minecraftdiamondsword big CNC rotated_v6 (Autodesk Fusion 360 design; units mm, degrees)
Autodesk Fusion 360 part; units mm, degrees
sketch "big huge diamond sword" plane through (0, 0, 0) normal (0, 0, 1) x (1, 0, 0)
  line L0 (0, 62.2254) -> (7.7782, 54.4472)
  line L1 (7.7782, 54.4472) -> (15.5563, 62.2254)
  line L2 (15.5563, 62.2254) -> (7.7782, 70.0036)
  line L3 (7.7782, 70.0036) -> (0, 62.2254)
  line L4 (7.7782, 54.4472) -> (15.5563, 46.669)
  line L5 (15.5563, 46.669) -> (23.3345, 54.4472)
  line L6 (23.3345, 54.4472) -> (15.5563, 62.2254)
  line L7 (15.5563, 62.2254) -> (7.7782, 54.4472)
  line L8 (15.5563, 46.669) -> (23.3345, 38.8909)
  line L9 (23.3345, 38.8909) -> (31.1127, 46.669)
  line L10 (23.3345, 54.4472) -> (15.5563, 46.669)
  line L11 (7.7782, 70.0036) -> (15.5563, 62.2254)
  line L12 (15.5563, 62.2254) -> (23.3345, 70.0036)
  line L13 (23.3345, 70.0036) -> (15.5563, 77.7817)
  line L14 (15.5563, 77.7817) -> (7.7782, 70.0036)
  line L15 (23.3345, 70.0036) -> (31.1127, 62.2254)
  line L16 (31.1127, 62.2254) -> (23.3345, 54.4472)
  line L17 (23.3345, 54.4472) -> (15.5563, 62.2254)
  line L18 (15.5563, 62.2254) -> (23.3345, 70.0036)
  line L19 (15.5563, 77.7817) -> (23.3345, 70.0036)
  line L20 (23.3345, 70.0036) -> (31.1127, 77.7817)
  line L21 (31.1127, 77.7817) -> (23.3345, 85.5599)
  line L22 (23.3345, 85.5599) -> (15.5563, 77.7817)
  line L23 (23.3345, 70.0036) -> (31.1127, 62.2254)
  line L24 (31.1127, 62.2254) -> (38.8909, 70.0036)
  line L25 (38.8909, 70.0036) -> (31.1127, 77.7817)
  line L26 (31.1127, 77.7817) -> (23.3345, 70.0036)
  line L27 (31.1127, 62.2254) -> (38.8909, 54.4472)
  line L28 (38.8909, 54.4472) -> (31.1127, 46.669)
  line L29 (31.1127, 46.669) -> (23.3345, 54.4472)
  line L30 (23.3345, 54.4472) -> (31.1127, 62.2254)
  line L31 (31.1127, 62.2254) -> (38.8909, 54.4472)
  line L32 (38.8909, 54.4472) -> (46.669, 62.2254)
  line L33 (46.669, 62.2254) -> (38.8909, 70.0036)
  line L34 (38.8909, 70.0036) -> (31.1127, 62.2254)
  line L35 (38.8909, 70.0036) -> (46.669, 62.2254)
  line L36 (46.669, 62.2254) -> (54.4472, 70.0036)
  line L37 (54.4472, 70.0036) -> (46.669, 77.7817)
  line L38 (46.669, 77.7817) -> (38.8909, 70.0036)
  line L39 (46.669, 62.2254) -> (54.4472, 54.4472)
  line L40 (54.4472, 54.4472) -> (46.669, 46.669)
  line L41 (46.669, 46.669) -> (38.8909, 54.4472)
  line L42 (38.8909, 54.4472) -> (46.669, 62.2254)
  line L43 (46.669, 62.2254) -> (54.4472, 54.4472)
  line L44 (54.4472, 54.4472) -> (62.2254, 62.2254)
  line L45 (62.2254, 62.2254) -> (54.4472, 70.0036)
  line L46 (54.4472, 70.0036) -> (46.669, 62.2254)
  line L47 (54.4472, 70.0036) -> (62.2254, 62.2254)
  line L48 (62.2254, 62.2254) -> (70.0036, 70.0036)
  line L49 (70.0036, 70.0036) -> (62.2254, 77.7817)
  line L50 (62.2254, 77.7817) -> (54.4472, 70.0036)
  line L51 (62.2254, 62.2254) -> (70.0036, 54.4472)
  line L52 (62.2254, 46.669) -> (54.4472, 54.4472)
  line L53 (54.4472, 54.4472) -> (62.2254, 62.2254)
  line L54 (62.2254, 62.2254) -> (70.0036, 54.4472)
  line L55 (70.0036, 54.4472) -> (77.7817, 62.2254)
  line L56 (77.7817, 62.2254) -> (70.0036, 70.0036)
  line L57 (70.0036, 70.0036) -> (62.2254, 62.2254)
  line L58 (70.0036, 70.0036) -> (77.7817, 62.2254)
  line L59 (77.7817, 62.2254) -> (85.5599, 70.0036)
  line L60 (85.5599, 70.0036) -> (77.7817, 77.7817)
  line L61 (77.7817, 77.7817) -> (70.0036, 70.0036)
  line L62 (77.7817, 77.7817) -> (70.0036, 85.5599)
  line L63 (70.0036, 85.5599) -> (77.7817, 93.3381)
  line L64 (77.7817, 93.3381) -> (85.5599, 85.5599)
  line L65 (85.5599, 85.5599) -> (77.7817, 77.7817)
  line L66 (77.7817, 93.3381) -> (85.5599, 85.5599)
  line L67 (85.5599, 85.5599) -> (93.3381, 93.3381)
  line L68 (93.3381, 93.3381) -> (85.5599, 101.1163)
  line L69 (85.5599, 101.1163) -> (77.7817, 93.3381)
  line L70 (85.5599, 101.1163) -> (77.7817, 108.8944)
  line L71 (77.7817, 108.8944) -> (85.5599, 116.6726)
  line L72 (85.5599, 116.6726) -> (93.3381, 108.8944)
  line L73 (93.3381, 108.8944) -> (85.5599, 101.1163)
  line L74 (85.5599, 116.6726) -> (93.3381, 108.8944)
  line L75 (93.3381, 108.8944) -> (101.1163, 116.6726)
  line L76 (101.1163, 116.6726) -> (93.3381, 124.4508)
  line L77 (93.3381, 124.4508) -> (85.5599, 116.6726)
  line L78 (93.3381, 108.8944) -> (101.1163, 101.1163)
  line L79 (101.1163, 101.1163) -> (108.8944, 108.8944)
  line L80 (108.8944, 108.8944) -> (101.1163, 116.6726)
  line L81 (101.1163, 116.6726) -> (93.3381, 108.8944)
  line L82 (85.5599, 101.1163) -> (93.3381, 93.3381)
  line L83 (93.3381, 93.3381) -> (101.1163, 101.1163)
  line L84 (101.1163, 101.1163) -> (93.3381, 108.8944)
  line L85 (93.3381, 108.8944) -> (85.5599, 101.1163)
  line L86 (101.1163, 101.1163) -> (108.8944, 93.3381)
  line L87 (108.8944, 93.3381) -> (101.1163, 85.5599)
  line L88 (101.1163, 85.5599) -> (93.3381, 93.3381)
  line L89 (93.3381, 93.3381) -> (101.1163, 101.1163)
  line L90 (93.3381, 93.3381) -> (101.1163, 85.5599)
  line L91 (101.1163, 85.5599) -> (93.3381, 77.7817)
  line L92 (93.3381, 77.7817) -> (85.5599, 85.5599)
  line L93 (85.5599, 85.5599) -> (93.3381, 93.3381)
  line L94 (77.7817, 77.7817) -> (85.5599, 70.0036)
  line L95 (85.5599, 70.0036) -> (93.3381, 77.7817)
  line L96 (93.3381, 77.7817) -> (85.5599, 85.5599)
  line L97 (85.5599, 85.5599) -> (77.7817, 77.7817)
  line L98 (70.0036, 54.4472) -> (77.7817, 46.669)
  line L99 (62.2254, 46.669) -> (70.0036, 54.4472)
  line L100 (77.7817, 62.2254) -> (85.5599, 54.4472)
  line L101 (85.5599, 54.4472) -> (77.7817, 46.669)
  line L102 (70.0036, 54.4472) -> (77.7817, 62.2254)
  line L103 (85.5599, 70.0036) -> (93.3381, 62.2254)
  line L104 (93.3381, 62.2254) -> (85.5599, 54.4472)
  line L105 (85.5599, 54.4472) -> (77.7817, 62.2254)
  line L106 (77.7817, 62.2254) -> (85.5599, 70.0036)
  line L107 (77.7817, 46.669) -> (85.5599, 38.8909)
  line L108 (85.5599, 38.8909) -> (77.7817, 31.1127)
  line L109 (77.7817, 31.1127) -> (70.0036, 38.8909)
  line L110 (70.0036, 38.8909) -> (77.7817, 46.669)
  line L111 (77.7817, 46.669) -> (85.5599, 38.8909)
  line L112 (85.5599, 38.8909) -> (93.3381, 46.669)
  line L113 (93.3381, 46.669) -> (85.5599, 54.4472)
  line L114 (85.5599, 54.4472) -> (77.7817, 46.669)
  line L115 (85.5599, 38.8909) -> (93.3381, 31.1127)
  line L116 (93.3381, 31.1127) -> (85.5599, 23.3345)
  line L117 (85.5599, 23.3345) -> (77.7817, 31.1127)
  line L118 (77.7817, 31.1127) -> (85.5599, 38.8909)
  line L119 (85.5599, 23.3345) -> (93.3381, 15.5563)
  line L120 (93.3381, 15.5563) -> (101.1163, 23.3345)
  line L121 (101.1163, 23.3345) -> (93.3381, 31.1127)
  line L122 (93.3381, 31.1127) -> (85.5599, 23.3345)
  line L123 (93.3381, 15.5563) -> (101.1163, 7.7782)
  line L124 (101.1163, 7.7782) -> (108.8944, 15.5563)
  line L125 (108.8944, 15.5563) -> (101.1163, 23.3345)
  line L126 (101.1163, 23.3345) -> (93.3381, 15.5563)
  line L127 (85.5599, 23.3345) -> (93.3381, 15.5563)
  line L128 (93.3381, 15.5563) -> (85.5599, 7.7782)
  line L129 (85.5599, 7.7782) -> (77.7817, 15.5563)
  line L130 (77.7817, 15.5563) -> (85.5599, 23.3345)
  line L131 (93.3381, 15.5563) -> (101.1163, 7.7782)
  line L132 (101.1163, 7.7782) -> (93.3381, 0)
  line L133 (93.3381, 0) -> (85.5599, 7.7782)
  line L134 (85.5599, 7.7782) -> (93.3381, 15.5563)
  line L135 (93.3381, 77.7817) -> (101.1163, 70.0036)
  line L136 (101.1163, 70.0036) -> (93.3381, 62.2254)
  line L137 (93.3381, 62.2254) -> (85.5599, 70.0036)
  line L138 (85.5599, 70.0036) -> (93.3381, 77.7817)
  line L139 (93.3381, 62.2254) -> (101.1163, 54.4472)
  line L140 (101.1163, 54.4472) -> (93.3381, 46.669)
  line L141 (93.3381, 46.669) -> (85.5599, 54.4472)
  line L142 (85.5599, 54.4472) -> (93.3381, 62.2254)
  line L143 (101.1163, 85.5599) -> (108.8944, 77.7817)
  line L144 (108.8944, 77.7817) -> (101.1163, 70.0036)
  line L145 (101.1163, 70.0036) -> (93.3381, 77.7817)
  line L146 (93.3381, 77.7817) -> (101.1163, 85.5599)
  line L147 (101.1163, 70.0036) -> (108.8944, 62.2254)
  line L148 (108.8944, 62.2254) -> (101.1163, 54.4472)
  line L149 (101.1163, 54.4472) -> (93.3381, 62.2254)
  line L150 (93.3381, 62.2254) -> (101.1163, 70.0036)
  line L151 (108.8944, 77.7817) -> (116.6726, 70.0036)
  line L152 (116.6726, 70.0036) -> (108.8944, 62.2254)
  line L153 (108.8944, 62.2254) -> (101.1163, 70.0036)
  line L154 (101.1163, 70.0036) -> (108.8944, 77.7817)
  line L155 (93.3381, 46.669) -> (101.1163, 38.8909)
  line L156 (101.1163, 38.8909) -> (93.3381, 31.1127)
  line L157 (93.3381, 31.1127) -> (85.5599, 38.8909)
  line L158 (85.5599, 38.8909) -> (93.3381, 46.669)
  line L159 (101.1163, 38.8909) -> (108.8944, 31.1127)
  line L160 (108.8944, 31.1127) -> (101.1163, 23.3345)
  line L161 (101.1163, 23.3345) -> (93.3381, 31.1127)
  line L162 (93.3381, 31.1127) -> (101.1163, 38.8909)
  line L163 (101.1163, 54.4472) -> (108.8944, 46.669)
  line L164 (108.8944, 46.669) -> (101.1163, 38.8909)
  line L165 (101.1163, 38.8909) -> (93.3381, 46.669)
  line L166 (93.3381, 46.669) -> (101.1163, 54.4472)
  line L167 (108.8944, 62.2254) -> (116.6726, 54.4472)
  line L168 (116.6726, 54.4472) -> (108.8944, 46.669)
  line L169 (108.8944, 46.669) -> (101.1163, 54.4472)
  line L170 (101.1163, 54.4472) -> (108.8944, 62.2254)
  line L171 (108.8944, 46.669) -> (101.1163, 54.4472)
  line L172 (101.1163, 54.4472) -> (108.8944, 62.2254)
  line L173 (108.8944, 62.2254) -> (116.6726, 54.4472)
  line L174 (116.6726, 54.4472) -> (108.8944, 46.669)
  line L175 (108.8944, 46.669) -> (116.6726, 38.8909)
  line L176 (116.6726, 38.8909) -> (124.4508, 46.669)
  line L177 (124.4508, 46.669) -> (116.6726, 54.4472)
  line L178 (116.6726, 54.4472) -> (108.8944, 46.669)
  line L179 (108.8944, 62.2254) -> (116.6726, 54.4472)
  line L180 (116.6726, 54.4472) -> (124.4508, 62.2254)
  line L181 (124.4508, 62.2254) -> (116.6726, 70.0036)
  line L182 (116.6726, 70.0036) -> (108.8944, 62.2254)
  line L183 (116.6726, 54.4472) -> (124.4508, 46.669)
  line L184 (124.4508, 46.669) -> (132.229, 54.4472)
  line L185 (132.229, 54.4472) -> (124.4508, 62.2254)
  line L186 (124.4508, 62.2254) -> (116.6726, 54.4472)
  line L187 (124.4508, 46.669) -> (132.229, 38.8909)
  line L188 (132.229, 38.8909) -> (140.0071, 46.669)
  line L189 (140.0071, 46.669) -> (132.229, 54.4472)
  line L190 (132.229, 54.4472) -> (124.4508, 46.669)
  line L191 (108.8944, 77.7817) -> (116.6726, 70.0036)
  line L192 (116.6726, 70.0036) -> (124.4508, 77.7817)
  line L193 (124.4508, 77.7817) -> (116.6726, 85.5599)
  line L194 (116.6726, 85.5599) -> (108.8944, 77.7817)
  line L195 (116.6726, 70.0036) -> (124.4508, 62.2254)
  line L196 (124.4508, 62.2254) -> (132.229, 70.0036)
  line L197 (132.229, 70.0036) -> (124.4508, 77.7817)
  line L198 (124.4508, 77.7817) -> (116.6726, 70.0036)
  line L199 (132.229, 70.0036) -> (124.4508, 77.7817)
  line L200 (124.4508, 77.7817) -> (132.229, 85.5599)
  line L201 (132.229, 85.5599) -> (140.0071, 77.7817)
  line L202 (140.0071, 77.7817) -> (132.229, 70.0036)
  line L203 (124.4508, 62.2254) -> (132.229, 54.4472)
  line L204 (132.229, 54.4472) -> (140.0071, 62.2254)
  line L205 (140.0071, 62.2254) -> (132.229, 70.0036)
  line L206 (132.229, 70.0036) -> (124.4508, 62.2254)
  line L207 (132.229, 70.0036) -> (140.0071, 62.2254)
  line L208 (140.0071, 62.2254) -> (147.7853, 70.0036)
  line L209 (147.7853, 70.0036) -> (140.0071, 77.7817)
  line L210 (140.0071, 77.7817) -> (132.229, 70.0036)
  line L211 (132.229, 54.4472) -> (140.0071, 46.669)
  line L212 (140.0071, 46.669) -> (147.7853, 54.4472)
  line L213 (147.7853, 54.4472) -> (140.0071, 62.2254)
  line L214 (140.0071, 62.2254) -> (132.229, 54.4472)
  line L215 (140.0071, 77.7817) -> (147.7853, 70.0036)
  line L216 (147.7853, 70.0036) -> (155.5635, 77.7817)
  line L217 (155.5635, 77.7817) -> (147.7853, 85.5599)
  line L218 (147.7853, 85.5599) -> (140.0071, 77.7817)
  line L219 (140.0071, 46.669) -> (147.7853, 38.8909)
  line L220 (147.7853, 38.8909) -> (155.5635, 46.669)
  line L221 (155.5635, 46.669) -> (147.7853, 54.4472)
  line L222 (147.7853, 54.4472) -> (140.0071, 46.669)
  line L223 (140.0071, 62.2254) -> (147.7853, 54.4472)
  line L224 (147.7853, 54.4472) -> (155.5635, 62.2254)
  line L225 (155.5635, 62.2254) -> (147.7853, 70.0036)
  line L226 (147.7853, 70.0036) -> (140.0071, 62.2254)
  line L227 (155.5635, 62.2254) -> (163.3417, 54.4472)
  line L228 (163.3417, 54.4472) -> (171.1198, 62.2254)
  line L229 (171.1198, 62.2254) -> (163.3417, 70.0036)
  line L230 (163.3417, 70.0036) -> (155.5635, 62.2254)
  line L231 (155.5635, 62.2254) -> (147.7853, 70.0036)
  line L232 (147.7853, 70.0036) -> (155.5635, 77.7817)
  line L233 (155.5635, 77.7817) -> (163.3417, 70.0036)
  line L234 (163.3417, 70.0036) -> (155.5635, 62.2254)
  line L235 (155.5635, 62.2254) -> (163.3417, 54.4472)
  line L236 (163.3417, 54.4472) -> (155.5635, 46.669)
  line L237 (155.5635, 46.669) -> (147.7853, 54.4472)
  line L238 (147.7853, 54.4472) -> (155.5635, 62.2254)
  line L239 (155.5635, 77.7817) -> (163.3417, 70.0036)
  line L240 (163.3417, 70.0036) -> (171.1198, 77.7817)
  line L241 (171.1198, 77.7817) -> (163.3417, 85.5599)
  line L242 (163.3417, 85.5599) -> (155.5635, 77.7817)
  line L243 (163.3417, 70.0036) -> (171.1198, 62.2254)
  line L244 (171.1198, 62.2254) -> (178.898, 70.0036)
  line L245 (178.898, 70.0036) -> (171.1198, 77.7817)
  line L246 (171.1198, 77.7817) -> (163.3417, 70.0036)
  line L247 (155.5635, 46.669) -> (163.3417, 38.8909)
  line L248 (163.3417, 38.8909) -> (171.1198, 46.669)
  line L249 (171.1198, 46.669) -> (163.3417, 54.4472)
  line L250 (163.3417, 54.4472) -> (155.5635, 46.669)
  line L251 (163.3417, 54.4472) -> (171.1198, 46.669)
  line L252 (171.1198, 46.669) -> (178.898, 54.4472)
  line L253 (178.898, 54.4472) -> (171.1198, 62.2254)
  line L254 (171.1198, 62.2254) -> (163.3417, 54.4472)
  line L255 (171.1198, 62.2254) -> (178.898, 54.4472)
  line L256 (178.898, 54.4472) -> (186.6762, 62.2254)
  line L257 (186.6762, 62.2254) -> (178.898, 70.0036)
  line L258 (178.898, 70.0036) -> (171.1198, 62.2254)
  line L259 (171.1198, 77.7817) -> (178.898, 70.0036)
  line L260 (178.898, 70.0036) -> (186.6762, 77.7817)
  line L261 (186.6762, 77.7817) -> (178.898, 85.5599)
  line L262 (178.898, 85.5599) -> (171.1198, 77.7817)
  line L263 (171.1198, 46.669) -> (178.898, 38.8909)
  line L264 (178.898, 38.8909) -> (186.6762, 46.669)
  line L265 (186.6762, 46.669) -> (178.898, 54.4472)
  line L266 (178.898, 54.4472) -> (171.1198, 46.669)
  line L267 (178.898, 70.0036) -> (186.6762, 62.2254)
  line L268 (186.6762, 62.2254) -> (194.4544, 70.0036)
  line L269 (194.4544, 70.0036) -> (186.6762, 77.7817)
  line L270 (186.6762, 77.7817) -> (178.898, 70.0036)
  line L271 (178.898, 54.4472) -> (186.6762, 46.669)
  line L272 (186.6762, 46.669) -> (194.4544, 54.4472)
  line L273 (194.4544, 54.4472) -> (186.6762, 62.2254)
  line L274 (186.6762, 62.2254) -> (178.898, 54.4472)
  line L275 (186.6762, 62.2254) -> (194.4544, 54.4472)
  line L276 (194.4544, 54.4472) -> (202.2325, 62.2254)
  line L277 (202.2325, 62.2254) -> (194.4544, 70.0036)
  line L278 (194.4544, 70.0036) -> (186.6762, 62.2254)
  line L279 (186.6762, 46.669) -> (194.4544, 38.8909)
  line L280 (194.4544, 38.8909) -> (202.2325, 46.669)
  line L281 (202.2325, 46.669) -> (194.4544, 54.4472)
  line L282 (194.4544, 54.4472) -> (186.6762, 46.669)
  line L283 (186.6762, 77.7817) -> (194.4544, 70.0036)
  line L284 (194.4544, 70.0036) -> (202.2325, 77.7817)
  line L285 (202.2325, 77.7817) -> (194.4544, 85.5599)
  line L286 (194.4544, 85.5599) -> (186.6762, 77.7817)
  line L287 (202.2325, 62.2254) -> (210.0107, 54.4472)
  line L288 (210.0107, 54.4472) -> (202.2325, 46.669)
  line L289 (202.2325, 46.669) -> (194.4544, 54.4472)
  line L290 (194.4544, 54.4472) -> (202.2325, 62.2254)
  line L291 (194.4544, 70.0036) -> (202.2325, 62.2254)
  line L292 (202.2325, 62.2254) -> (210.0107, 70.0036)
  line L293 (210.0107, 70.0036) -> (202.2325, 77.7817)
  line L294 (202.2325, 77.7817) -> (194.4544, 70.0036)
  line L295 (202.2325, 62.2254) -> (210.0107, 54.4472)
  line L296 (210.0107, 54.4472) -> (217.7889, 62.2254)
  line L297 (217.7889, 62.2254) -> (210.0107, 70.0036)
  line L298 (210.0107, 70.0036) -> (202.2325, 62.2254)
  line L299 (202.2325, 46.669) -> (210.0107, 38.8909)
  line L300 (210.0107, 38.8909) -> (217.7889, 46.669)
  line L301 (217.7889, 46.669) -> (210.0107, 54.4472)
  line L302 (210.0107, 54.4472) -> (202.2325, 46.669)
  line L303 (202.2325, 77.7817) -> (210.0107, 70.0036)
  line L304 (210.0107, 70.0036) -> (217.7889, 77.7817)
  line L305 (217.7889, 77.7817) -> (210.0107, 85.5599)
  line L306 (210.0107, 85.5599) -> (202.2325, 77.7817)
  line L307 (217.7889, 77.7817) -> (225.5671, 70.0036)
  line L308 (225.5671, 70.0036) -> (217.7889, 62.2254)
  line L309 (217.7889, 62.2254) -> (210.0107, 70.0036)
  line L310 (210.0107, 70.0036) -> (217.7889, 77.7817)
  line L311 (210.0107, 54.4472) -> (217.7889, 46.669)
  line L312 (217.7889, 46.669) -> (225.5671, 54.4472)
  line L313 (225.5671, 54.4472) -> (217.7889, 62.2254)
  line L314 (217.7889, 62.2254) -> (210.0107, 54.4472)
  line L315 (217.7889, 62.2254) -> (225.5671, 54.4472)
  line L316 (225.5671, 54.4472) -> (233.3452, 62.2254)
  line L317 (233.3452, 62.2254) -> (225.5671, 70.0036)
  line L318 (225.5671, 70.0036) -> (217.7889, 62.2254)
  line L319 (217.7889, 77.7817) -> (225.5671, 70.0036)
  line L320 (225.5671, 70.0036) -> (233.3452, 77.7817)
  line L321 (233.3452, 77.7817) -> (225.5671, 85.5599)
  line L322 (225.5671, 85.5599) -> (217.7889, 77.7817)
  line L323 (225.5671, 70.0036) -> (233.3452, 62.2254)
  line L324 (233.3452, 62.2254) -> (241.1234, 70.0036)
  line L325 (241.1234, 70.0036) -> (233.3452, 77.7817)
  line L326 (233.3452, 77.7817) -> (225.5671, 70.0036)
  line L327 (217.7889, 46.669) -> (225.5671, 38.8909)
  line L328 (225.5671, 38.8909) -> (233.3452, 46.669)
  line L329 (233.3452, 46.669) -> (225.5671, 54.4472)
  line L330 (225.5671, 54.4472) -> (217.7889, 46.669)
  line L331 (225.5671, 54.4472) -> (233.3452, 46.669)
  line L332 (233.3452, 46.669) -> (241.1234, 54.4472)
  line L333 (241.1234, 54.4472) -> (233.3452, 62.2254)
  line L334 (233.3452, 62.2254) -> (225.5671, 54.4472)
  line L335 (233.3452, 62.2254) -> (225.5671, 70.0036)
  line L336 (225.5671, 70.0036) -> (233.3452, 77.7817)
  line L337 (233.3452, 77.7817) -> (241.1234, 70.0036)
  line L338 (241.1234, 70.0036) -> (233.3452, 62.2254)
  line L339 (233.3452, 62.2254) -> (241.1234, 54.4472)
  line L340 (241.1234, 54.4472) -> (248.9016, 62.2254)
  line L341 (248.9016, 62.2254) -> (241.1234, 70.0036)
  line L342 (241.1234, 70.0036) -> (233.3452, 62.2254)
  circle A0 centre (10, 10) radius 2.05
  circle A1 centre (200, 10) radius 2.05
  line L343 (0, 62.2254) -> (248.9016, 62.2254) construction
  circle A2 centre (200, 114.4508) radius 2.05
  point P0 (10, 114.4508)
  dimension "d249" = 11
  dimension "d250" = 11
  dimension "d251" = 11
  dimension "d252" = 11
  dimension "d253" = 11
  dimension "d254" = 11
  dimension "d255" = 11
  dimension "d256" = 11
  dimension "d261" = 11
  dimension "d262" = 11
  dimension "d263" = 11
  dimension "d264" = 11
  dimension "d265" = 11
  dimension "d266" = 11
  dimension "d267" = 11
  dimension "d268" = 11
  dimension "d271" = 11
  dimension "d272" = 11
  dimension "d273" = 11
  dimension "d274" = 11
  dimension "d275" = 11
  dimension "d276" = 11
  dimension "d277" = 11
  dimension "d278" = 11
  dimension "d279" = 11
  dimension "d280" = 11
  dimension "d281" = 11
  dimension "d282" = 11
  dimension "d283" = 11
  dimension "d284" = 11
  dimension "d285" = 11
  dimension "d286" = 11
  dimension "d287" = 11
  dimension "d288" = 11
  dimension "d289" = 11
  dimension "d290" = 11
  dimension "d291" = 11
  dimension "d292" = 11
  dimension "d293" = 11
  dimension "d294" = 11
  dimension "d295" = 11
  dimension "d296" = 11
  dimension "d297" = 11
  dimension "d298" = 11
  dimension "d299" = 11
  dimension "d300" = 11
  dimension "d301" = 11
  dimension "d302" = 11
  dimension "d303" = 11
  dimension "d304" = 11
  dimension "d309" = 11
  dimension "d310" = 11
  dimension "d311" = 11
  dimension "d312" = 11
  dimension "d313" = 11
  dimension "d314" = 11
  dimension "d315" = 11
  dimension "d316" = 11
  dimension "d319" = 11
  dimension "d320" = 11
  dimension "d321" = 11
  dimension "d322" = 11
  dimension "d323" = 11
  dimension "d324" = 11
  dimension "d325" = 11
  dimension "d326" = 11
  dimension "d327" = 11
  dimension "d328" = 11
  dimension "d329" = 11
  dimension "d330" = 11
  dimension "d331" = 11
  dimension "d332" = 11
  dimension "d333" = 11
  dimension "d334" = 11
  dimension "d335" = 11
  dimension "d336" = 11
  dimension "d337" = 11
  dimension "d338" = 11
  dimension "d339" = 11
  dimension "d340" = 11
  dimension "d341" = 11
  dimension "d342" = 11
  dimension "d343" = 11
  dimension "d344" = 11
  dimension "d345" = 11
  dimension "d346" = 11
  dimension "d347" = 11
  dimension "d348" = 11
  dimension "d349" = 11
  dimension "d350" = 11
  dimension "d351" = 11
  dimension "d352" = 11
  dimension "d353" = 11
  dimension "d354" = 11
  dimension "d355" = 11
  dimension "d356" = 11
  dimension "d357" = 11
  dimension "d358" = 11
  dimension "d359" = 11
  dimension "d360" = 11
  dimension "d361" = 11
  dimension "d362" = 11
  dimension "d363" = 11
  dimension "d364" = 11
  dimension "d365" = 11
  dimension "d366" = 11
  dimension "d367" = 11
  dimension "d368" = 11
  dimension "d369" = 11
  dimension "d370" = 11
  dimension "d371" = 11
  dimension "d372" = 11
  dimension "d373" = 11
  dimension "d374" = 11
  dimension "d375" = 11
  dimension "d376" = 11
  dimension "d377" = 11
  dimension "d378" = 11
  dimension "d379" = 11
  dimension "d380" = 11
  dimension "d381" = 11
  dimension "d382" = 11
  dimension "d383" = 11
  dimension "d384" = 11
  dimension "d385" = 11
  dimension "d386" = 11
  dimension "d387" = 11
  dimension "d388" = 11
  dimension "d389" = 11
  dimension "d390" = 11
  dimension "d391" = 11
  dimension "d392" = 11
  dimension "d393" = 11
  dimension "d394" = 11
  dimension "d395" = 11
  dimension "d396" = 11
  dimension "d397" = 11
  dimension "d398" = 11
  dimension "d399" = 11
  dimension "d400" = 11
  dimension "d401" = 11
  dimension "d402" = 11
  dimension "d403" = 11
  dimension "d404" = 11
  dimension "d405" = 11
  dimension "d406" = 11
  dimension "d407" = 11
  dimension "d408" = 11
  dimension "d409" = 11
  dimension "d410" = 11
  dimension "d411" = 11
  dimension "d412" = 11
  dimension "d413" = 11
  dimension "d414" = 11
  dimension "d415" = 11
  dimension "d416" = 11
  dimension "d417" = 11
  dimension "d418" = 11
  dimension "d419" = 11
  dimension "d420" = 11
  dimension "d421" = 11
  dimension "d422" = 11
  dimension "d423" = 11
  dimension "d424" = 11
  dimension "d425" = 11
  dimension "d426" = 11
  dimension "d427" = 11
  dimension "d428" = 11
  dimension "d429" = 11
  dimension "d430" = 11
  dimension "d431" = 11
  dimension "d432" = 11
  dimension "d433" = 11
  dimension "d434" = 11
  dimension "d453" = 4.1
  dimension "d454" = 4.1
  dimension "d455" = 10
  dimension "d456" = 200
  dimension "d457" = 10
  constraint perpendicular L74 L75
  constraint parallel L75 L77
  constraint perpendicular L78 L79
  constraint parallel L79 L81
  constraint perpendicular L86 L87
  constraint parallel L87 L89
  constraint perpendicular L103 L104
  constraint parallel L104 L106
  constraint perpendicular L52 L99
  constraint coincident L98.end L101.end
  constraint perpendicular L115 L116
  constraint parallel L116 L118
  constraint perpendicular L123 L124
  constraint parallel L124 L126
  constraint perpendicular L127 L128
  constraint parallel L128 L130
  constraint perpendicular L131 L132
  constraint parallel L132 L134
  constraint perpendicular L135 L136
  constraint parallel L136 L138
  constraint perpendicular L139 L140
  constraint parallel L140 L142
  constraint perpendicular L143 L144
  constraint parallel L144 L146
  constraint perpendicular L147 L148
  constraint parallel L148 L150
  constraint perpendicular L151 L152
  constraint parallel L152 L154
  constraint perpendicular L155 L156
  constraint parallel L156 L158
  constraint perpendicular L159 L160
  constraint parallel L160 L162
  constraint perpendicular L163 L164
  constraint parallel L164 L166
  constraint perpendicular L167 L168
  constraint parallel L168 L170
  constraint perpendicular L171 L172
  constraint parallel L172 L174
  constraint perpendicular L175 L176
  constraint parallel L176 L178
  constraint perpendicular L179 L180
  constraint parallel L180 L182
  constraint perpendicular L183 L184
  constraint parallel L184 L186
  constraint perpendicular L187 L188
  constraint parallel L188 L190
  constraint perpendicular L195 L196
  constraint parallel L196 L198
  constraint perpendicular L199 L200
  constraint parallel L200 L202
  constraint perpendicular L203 L204
  constraint parallel L204 L206
  constraint perpendicular L211 L212
  constraint parallel L212 L214
  constraint perpendicular L215 L216
  constraint parallel L216 L218
  constraint perpendicular L219 L220
  constraint parallel L220 L222
  constraint perpendicular L223 L224
  constraint parallel L224 L226
  constraint perpendicular L227 L228
  constraint parallel L228 L230
  constraint perpendicular L231 L232
  constraint parallel L232 L234
  constraint perpendicular L235 L236
  constraint parallel L236 L238
  constraint perpendicular L239 L240
  constraint parallel L240 L242
  constraint perpendicular L243 L244
  constraint parallel L244 L246
  constraint perpendicular L247 L248
  constraint parallel L248 L250
  constraint perpendicular L251 L252
  constraint parallel L252 L254
  constraint perpendicular L255 L256
  constraint parallel L256 L258
  constraint perpendicular L259 L260
  constraint parallel L260 L262
  constraint perpendicular L263 L264
  constraint parallel L264 L266
  constraint perpendicular L267 L268
  constraint parallel L268 L270
  constraint perpendicular L275 L276
  constraint parallel L276 L278
  constraint perpendicular L279 L280
  constraint parallel L280 L282
  constraint perpendicular L283 L284
  constraint parallel L284 L286
  constraint perpendicular L287 L288
  constraint parallel L288 L290
  constraint perpendicular L291 L292
  constraint parallel L292 L294
  constraint perpendicular L303 L304
  constraint parallel L304 L306
  constraint perpendicular L339 L340
  constraint parallel L340 L342
  constraint horizontal A0.centre A1.centre
  constraint symmetric A0.centre L343 P0
  constraint symmetric A1 L343 A2
  measures "d249" distance of L0.start L0.end
  measures "d250" distance of L0.start L2.end
  measures "d251" distance of L0.end L4.end
  measures "d252" distance of L0.end L1.end
  measures "d253" distance of L4.end L8.end
  measures "d254" distance of L4.end L5.end
  measures "d255" distance of L2.end L1.end
  measures "d256" distance of L2.end L13.end
  measures "d261" distance of L12.end L15.end
  measures "d262" distance of L12.end L1.end
  measures "d263" distance of L13.end L12.end
  measures "d264" distance of L13.end L21.end
  measures "d265" distance of L12.end L15.end
  measures "d266" distance of L12.end L20.end
  measures "d267" distance of L15.end L27.end
  measures "d268" distance of L15.end L5.end
  measures "d271" distance of L15.end L27.end
  measures "d272" distance of L15.end L24.end
  measures "d273" distance of L24.end L32.end
  measures "d274" distance of L24.end L37.end
  measures "d275" distance of L32.end L39.end
  measures "d276" distance of L32.end L27.end
  measures "d277" distance of L32.end L39.end
  measures "d278" distance of L32.end L36.end
  measures "d279" distance of L36.end L44.end
  measures "d280" distance of L36.end L49.end
  measures "d281" distance of L44.end L51.end
  measures "d282" distance of L44.end L39.end
  measures "d283" distance of L44.end L51.end
  measures "d284" distance of L44.end L48.end
  measures "d285" distance of L48.end L55.end
  measures "d286" distance of L48.end L60.end
  measures "d287" distance of L60.end L62.end
  measures "d288" distance of L60.end L64.end
  measures "d289" distance of L63.end L64.end
  measures "d290" distance of L63.end L68.end
  measures "d291" distance of L68.end L70.end
  measures "d292" distance of L68.end L72.end
  measures "d293" distance of L71.end L72.end
  measures "d294" distance of L71.end L76.end
  measures "d295" distance of L72.end L78.end
  measures "d296" distance of L72.end L75.end
  measures "d297" distance of L68.end L67.end
  measures "d298" distance of L68.end L72.end
  measures "d299" distance of L78.end L86.end
  measures "d300" distance of L78.end L67.end
  measures "d301" distance of L67.end L87.end
  measures "d302" distance of L67.end L64.end
  measures "d303" distance of L60.end L59.end
  measures "d304" distance of L60.end L64.end
  measures "d309" distance of L51.end L98.end
  measures "d310" distance of L51.end L52.start
  measures "d311" distance of L55.end L100.end
  measures "d312" distance of L55.end L51.end
  measures "d313" distance of L59.end L103.end
  measures "d314" distance of L59.end L55.end
  measures "d315" distance of L98.end L107.end
  measures "d316" distance of L98.end L109.end
  measures "d319" distance of L98.end L107.end
  measures "d320" distance of L98.end L100.end
  measures "d321" distance of L107.end L115.end
  measures "d322" distance of L107.end L108.end
  measures "d323" distance of L116.end L119.end
  measures "d324" distance of L116.end L115.end
  measures "d325" distance of L119.end L123.end
  measures "d326" distance of L119.end L120.end
  measures "d327" distance of L116.end L119.end
  measures "d328" distance of L116.end L129.end
  measures "d329" distance of L119.end L123.end
  measures "d330" distance of L119.end L128.end
  measures "d331" distance of L91.end L135.end
  measures "d332" distance of L91.end L59.end
  measures "d333" distance of L103.end L139.end
  measures "d334" distance of L103.end L100.end
  measures "d335" distance of L87.end L143.end
  measures "d336" distance of L87.end L91.end
  measures "d337" distance of L135.end L147.end
  measures "d338" distance of L135.end L103.end
  measures "d339" distance of L143.end L151.end
  measures "d340" distance of L143.end L135.end
  measures "d341" distance of L112.end L155.end
  measures "d342" distance of L112.end L107.end
  measures "d343" distance of L155.end L159.end
  measures "d344" distance of L155.end L115.end
  measures "d345" distance of L139.end L163.end
  measures "d346" distance of L139.end L112.end
  measures "d347" distance of L147.end L167.end
  measures "d348" distance of L147.end L139.end
  measures "d349" distance of L163.end L139.end
  measures "d350" distance of L163.end L167.end
  measures "d351" distance of L163.end L175.end
  measures "d352" distance of L163.end L167.end
  measures "d353" distance of L147.end L167.end
  measures "d354" distance of L147.end L151.end
  measures "d355" distance of L167.end L176.end
  measures "d356" distance of L167.end L180.end
  measures "d357" distance of L176.end L187.end
  measures "d358" distance of L176.end L184.end
  measures "d359" distance of L143.end L151.end
  measures "d360" distance of L143.end L193.end
  measures "d361" distance of L151.end L180.end
  measures "d362" distance of L151.end L192.end
  measures "d363" distance of L196.end L192.end
  measures "d364" distance of L196.end L201.end
  measures "d365" distance of L180.end L184.end
  measures "d366" distance of L180.end L196.end
  measures "d367" distance of L196.end L204.end
  measures "d368" distance of L196.end L201.end
  measures "d369" distance of L184.end L188.end
  measures "d370" distance of L184.end L204.end
  measures "d371" distance of L201.end L208.end
  measures "d372" distance of L201.end L217.end
  measures "d373" distance of L188.end L219.end
  measures "d374" distance of L188.end L212.end
  measures "d375" distance of L204.end L212.end
  measures "d376" distance of L204.end L208.end
  measures "d377" distance of L224.end L227.end
  measures "d378" distance of L224.end L229.end
  measures "d379" distance of L224.end L208.end
  measures "d380" distance of L224.end L229.end
  measures "d381" distance of L224.end L227.end
  measures "d382" distance of L224.end L212.end
  measures "d383" distance of L216.end L229.end
  measures "d384" distance of L216.end L241.end
  measures "d385" distance of L229.end L228.end
  measures "d386" distance of L229.end L240.end
  measures "d387" distance of L220.end L247.end
  measures "d388" distance of L220.end L227.end
  measures "d389" distance of L227.end L248.end
  measures "d390" distance of L227.end L228.end
  measures "d391" distance of L228.end L252.end
  measures "d392" distance of L228.end L244.end
  measures "d393" distance of L240.end L244.end
  measures "d394" distance of L240.end L261.end
  measures "d395" distance of L248.end L263.end
  measures "d396" distance of L248.end L252.end
  measures "d397" distance of L244.end L256.end
  measures "d398" distance of L244.end L260.end
  measures "d399" distance of L252.end L264.end
  measures "d400" distance of L252.end L256.end
  measures "d401" distance of L256.end L272.end
  measures "d402" distance of L256.end L268.end
  measures "d403" distance of L264.end L279.end
  measures "d404" distance of L264.end L272.end
  measures "d405" distance of L260.end L268.end
  measures "d406" distance of L260.end L285.end
  measures "d407" distance of L276.end L287.end
  measures "d408" distance of L276.end L272.end
  measures "d409" distance of L268.end L276.end
  measures "d410" distance of L268.end L284.end
  measures "d411" distance of L276.end L287.end
  measures "d412" distance of L276.end L292.end
  measures "d413" distance of L280.end L299.end
  measures "d414" distance of L280.end L287.end
  measures "d415" distance of L284.end L292.end
  measures "d416" distance of L284.end L305.end
  measures "d417" distance of L304.end L307.end
  measures "d418" distance of L304.end L292.end
  measures "d419" distance of L287.end L300.end
  measures "d420" distance of L287.end L296.end
  measures "d421" distance of L296.end L312.end
  measures "d422" distance of L296.end L307.end
  measures "d423" distance of L304.end L307.end
  measures "d424" distance of L304.end L321.end
  measures "d425" distance of L307.end L316.end
  measures "d426" distance of L307.end L320.end
  measures "d427" distance of L300.end L327.end
  measures "d428" distance of L300.end L312.end
  measures "d429" distance of L312.end L328.end
  measures "d430" distance of L312.end L316.end
  measures "d431" distance of L316.end L307.end
  measures "d432" distance of L316.end L324.end
  measures "d433" distance of L316.end L332.end
  measures "d434" distance of L316.end L324.end
  measures "d453" diameter of A0
  measures "d454" diameter of A1
  measures "d455" horizontal distance of origin A0.centre
  measures "d456" horizontal distance of origin A1.centre
  measures "d457" vertical distance of A1.centre origin
sketch "board prepare" plane through (0, 0, 0) normal (0, 0, 1) x (1, 0, 0)
  line L0 (219.2031, -219.2031) -> (306.8843, -131.5219)
  dimension "d437" = 310
  measures "d437" distance of origin L0.start
extrude "Extrude13" add sketch "big huge diamond sword" along normal blind 23 contours L0 L1 L2 L3 L7 L11 | L1 L4 L5 L6 L7 L10 L17 | L2 L11 L12 L13 L14 L18 L19 | L6 L12 L15 L16 L17 L18 L23 L30 | L5 L8 L9 L10 L29 | L13 L19 L20 L21 L22 L26 | L16 L27 L28 L29 L30 L31 | L15 L20 L23 L24 L25 L26 L34 | L24 L27 L31 L32 L33 L34 L35 L42 | L33 L35 L36 L37 L38 L46 | L32 L39 L40 L41 L42 L43 | L36 L39 L43 L44 L45 L46 L47 L53 | L45 L47 L48 L49 L50 L57 | L44 L51 L52 L53 L54 L99 | L48 L51 L54 L55 L56 L57 L58 L102 | L56 L58 L59 L60 L61 L94 L106 | L55 L98 L100 L101 L102 L105 L114 | L59 L100 L103 L104 L105 L106 L137 L142 | L60 L65 L92 L94 L95 L96 L97 L138 | L62 L63 L64 L65 L66 L97 | L101 L107 L111 L112 L113 L114 L141 L158 | L107 L108 L109 L110 L111 L118 | L95 L103 L135 L136 L137 L138 L145 L150 | L104 L113 L139 L140 L141 L142 L149 L166 | L64 L66 L67 L68 L69 L82 L93 | L67 L88 L90 L91 L92 L93 L96 L146 | L108 L115 L116 L117 L118 L122 L157 | L112 L115 L155 L156 L157 L158 L162 L165 | L91 L135 L143 L144 L145 L146 L154 | L136 L139 L147 L148 L149 L150 L153 L170 L172 | L140 L155 L163 L164 L165 L166 L169 L171 | L68 L73 L78 L82 L83 L84 L85 L89 | L83 L86 L87 L88 L89 L90 | L116 L119 L120 L121 L122 L126 L127 L161 | L121 L156 L159 L160 L161 L162 | L144 L147 L151 L152 L153 L154 L182 L191 | L148 L163 L167 L168 L169 L170 L171 L172 L173 L174 L178 L179 | L70 L71 L72 L73 L74 L85 | L75 L78 L79 L80 L81 L84 | L119 L127 L128 L129 L130 L134 | L120 L123 L124 L125 L126 L131 | L151 L191 L192 L193 L194 L198 | L152 L167 L173 L179 L180 L181 L182 L186 L195 | L168 L174 L175 L176 L177 L178 L183 | L72 L74 L75 L76 L77 L81 | L123 L128 L131 L132 L133 L134 | L181 L192 L195 L196 L197 L198 L199 L206 | L177 L180 L183 L184 L185 L186 L190 L203 | L185 L196 L203 L204 L205 L206 L207 L214 | L197 L199 L200 L201 L202 L210 | L184 L187 L188 L189 L190 L211 | L189 L204 L211 L212 L213 L214 L222 L223 | L202 L205 L207 L208 L209 L210 L215 L226 | L212 L219 L220 L221 L222 L237 | L208 L213 L223 L224 L225 L226 L231 L238 | L209 L215 L216 L217 L218 L232 | L221 L224 L227 L235 L236 L237 L238 L250 | L216 L225 L230 L231 L232 L233 L234 L239 | L236 L247 L248 L249 L250 L251 | L227 L228 L229 L230 L234 L235 L243 L254 | L233 L239 L240 L241 L242 L246 | L228 L249 L251 L252 L253 L254 L255 L266 | L229 L240 L243 L244 L245 L246 L258 L259 | L244 L253 L255 L256 L257 L258 L267 L274 | L252 L263 L264 L265 L266 L271 | L245 L259 L260 L261 L262 L270 | L257 L260 L267 L268 L269 L270 L278 L283 | L256 L265 L271 L272 L273 L274 L275 L282 | L268 L273 L275 L276 L277 L278 L290 L291 | L269 L283 L284 L285 L286 L294 | L272 L279 L280 L281 L282 L289 | L277 L284 L291 L292 L293 L294 L298 L303 | L276 L281 L287 L288 L289 L290 L295 L302 | L287 L292 L295 L296 L297 L298 L309 L314 | L293 L303 L304 L305 L306 L310 | L288 L299 L300 L301 L302 L311 | L296 L301 L311 L312 L313 L314 L315 L330 | L297 L304 L307 L308 L309 L310 L318 L319 | L308 L313 L315 L316 L317 L318 L323 L334 L335 | L312 L327 L328 L329 L330 L331 | L307 L319 L320 L321 L322 L326 L336 | L317 L320 L323 L324 L325 L326 L335 L336 L337 L338 L342 | L316 L329 L331 L332 L333 L334 L339 | L324 L333 L338 L339 L340 L341 L342
equation "d = 11 mm"
equation "StockHeight = 23 mm"
equation "d249 = d"
equation "d250 = d"
equation "d251 = d"
equation "d252 = d"
equation "d253 = d"
equation "d254 = d"
equation "d255 = d"
equation "d256 = d"
equation "d261 = d"
equation "d262 = d"
equation "d263 = d"
equation "d264 = d"
equation "d265 = d"
equation "d266 = d"
equation "d267 = d"
equation "d268 = d"
equation "d271 = d"
equation "d272 = d"
equation "d273 = d"
equation "d274 = d"
equation "d275 = d"
equation "d276 = d"
equation "d277 = d"
equation "d278 = d"
equation "d279 = d"
equation "d280 = d"
equation "d281 = d"
equation "d282 = d"
equation "d283 = d"
equation "d284 = d"
equation "d285 = d"
equation "d286 = d"
equation "d287 = d"
equation "d288 = d"
equation "d289 = d"
equation "d290 = d"
equation "d291 = d"
equation "d292 = d"
equation "d293 = d"
equation "d294 = d"
equation "d295 = d"
equation "d296 = d"
equation "d297 = d"
equation "d298 = d"
equation "d299 = d"
equation "d300 = d"
equation "d301 = d"
equation "d302 = d"
equation "d303 = d"
equation "d304 = d"
equation "d309 = d"
equation "d310 = d"
equation "d311 = d"
equation "d312 = d"
equation "d313 = d"
equation "d314 = d"
equation "d315 = d"
equation "d316 = d"
equation "d319 = d"
equation "d320 = d"
equation "d321 = d"
equation "d322 = d"
equation "d323 = d"
equation "d324 = d"
equation "d325 = d"
equation "d326 = d"
equation "d327 = d"
equation "d328 = d"
equation "d329 = d"
equation "d330 = d"
equation "d331 = d"
equation "d332 = d"
equation "d333 = d"
equation "d334 = d"
equation "d335 = d"
equation "d336 = d"
equation "d337 = d"
equation "d338 = d"
equation "d339 = d"
equation "d340 = d"
equation "d341 = d"
equation "d342 = d"
equation "d343 = d"
equation "d344 = d"
equation "d345 = d"
equation "d346 = d"
equation "d347 = d"
equation "d348 = d"
equation "d349 = d"
equation "d350 = d"
equation "d351 = d"
equation "d352 = d"
equation "d353 = d"
equation "d354 = d"
equation "d355 = d"
equation "d356 = d"
equation "d357 = d"
equation "d358 = d"
equation "d359 = d"
equation "d360 = d"
equation "d361 = d"
equation "d362 = d"
equation "d363 = d"
equation "d364 = d"
equation "d365 = d"
equation "d366 = d"
equation "d367 = d"
equation "d368 = d"
equation "d369 = d"
equation "d370 = d"
equation "d371 = d"
equation "d372 = d"
equation "d373 = d"
equation "d374 = d"
equation "d375 = d"
equation "d376 = d"
equation "d377 = d"
equation "d378 = d"
equation "d379 = d"
equation "d380 = d"
equation "d381 = d"
equation "d382 = d"
equation "d383 = d"
equation "d384 = d"
equation "d385 = d"
equation "d386 = d"
equation "d387 = d"
equation "d388 = d"
equation "d389 = d"
equation "d390 = d"
equation "d391 = d"
equation "d392 = d"
equation "d393 = d"
equation "d394 = d"
equation "d395 = d"
equation "d396 = d"
equation "d397 = d"
equation "d398 = d"
equation "d399 = d"
equation "d400 = d"
equation "d401 = d"
equation "d402 = d"
equation "d403 = d"
equation "d404 = d"
equation "d405 = d"
equation "d406 = d"
equation "d407 = d"
equation "d408 = d"
equation "d409 = d"
equation "d410 = d"
equation "d411 = d"
equation "d412 = d"
equation "d413 = d"
equation "d414 = d"
equation "d415 = d"
equation "d416 = d"
equation "d417 = d"
equation "d418 = d"
equation "d419 = d"
equation "d420 = d"
equation "d421 = d"
equation "d422 = d"
equation "d423 = d"
equation "d424 = d"
equation "d425 = d"
equation "d426 = d"
equation "d427 = d"
equation "d428 = d"
equation "d429 = d"
equation "d430 = d"
equation "d431 = d"
equation "d432 = d"
equation "d433 = d"
equation "d434 = d"
named bodies: "sword"
